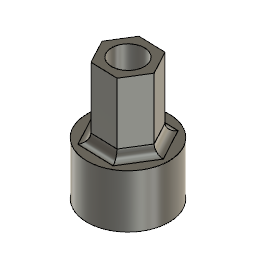
tt_motor_axle_adapter_6mm (Autodesk Fusion 360 design; units mm, degrees)
part number: 2026-02-17-20-52-45-499
Autodesk Fusion 360 part; units mm, degrees
sketch "Skizze1" plane through (0, 0, 0) normal (0, 0, 1) x (1, 0, 0)
  circle A0 centre (0, 0) radius 2.8
  circle A1 centre (0, 0) radius 5
  line L0 (1.95, -2.0094) -> (-1.95, -2.0094)
  line L1 (-1.95, -2.0094) -> (-1.95, 2.0094)
  line L2 (-1.95, 2.0094) -> (1.95, 2.0094)
  line L3 (1.95, 2.0094) -> (1.95, -2.0094)
  line L4 (1.95, -2.0094) -> (-1.95, 2.0094) construction
  line L5 (-1.95, -2.0094) -> (1.95, 2.0094) construction
  dimension "d1" = 5.6
  dimension "d2" = 10
  dimension "d3" = 3.9
  constraint coincident A0.centre A1.centre
  constraint horizontal L0
  constraint perpendicular L0 L1
  constraint parallel L0 L2
  constraint parallel L1 L3
  constraint coincident L4 A0.centre
  constraint coincident L5 A0.centre
  constraint coincident A0 L1.end
  measures "d1" diameter of A0
  measures "d2" diameter of A1
  measures "d3" distance of L1.end L2.end
extrude "Extrusion1" add sketch "Skizze1" along normal blind 6.5 contours A0 L3 | A0 L1 | A1 makes body 1
ref_plane "Arbeitsebene1" through (0, 0, 6.5) normal (0, 0, 1) x (1, 0, 0)
sketch "Skizze2" plane through (0, 0, 6.5) normal (0, 0, 1) x (1, 0, 0)
  line L0 (-3.2893, 0.101) -> (-1.7322, -2.7981)
  line L1 (-1.7322, -2.7981) -> (1.5572, -2.8992)
  line L2 (1.5572, -2.8992) -> (3.2893, -0.101)
  line L3 (3.2893, -0.101) -> (1.7322, 2.7981)
  line L4 (1.7322, 2.7981) -> (-1.5572, 2.8992)
  line L5 (-1.5572, 2.8992) -> (-3.2893, 0.101)
  dimension "d7" = 2.85
  measures "d7" distance of origin L5
extrude "Extrusion2" add sketch "Skizze2" along normal blind 10.5 separate body makes body 2
sketch "Skizze3" plane through (0, 0, 17) normal (0, 0, 1) x (-1, 0, 0)
  line L0 (1.5572, -2.8992) -> (3.2893, -0.101)
  line L1 (3.2893, -0.101) -> (1.7322, 2.7981)
  line L2 (1.7322, 2.7981) -> (-1.5572, 2.8992)
  line L3 (-1.5572, 2.8992) -> (-3.2893, 0.101)
  line L4 (-3.2893, 0.101) -> (-1.7322, -2.7981)
  line L5 (-1.7322, -2.7981) -> (1.5572, -2.8992)
  circle A0 centre (0, 0) radius 2
  dimension "d10" = 4
  constraint coincident A0.centre origin
  measures "d10" diameter of A0
extrude "Extrusion3" cut sketch "Skizze3" against normal blind 10.5 contours A0 bodies 2
combine "Kombinieren1" operation add target body 1 tool bodies 2
fillet "Abrundung1" radius 1 6 edges at (2.4233, -1.5001, 6.5) (2.5108, 1.3485, 6.5) (0.0875, 2.8487, 6.5) (-0.0875, -2.8487, 6.5) (-2.5108, -1.3485, 6.5) (-2.4233, 1.5001, 6.5) on bodies 1
extrude "Extrusion4" cut 1 faces at (-0.1082, -2.5639, 17) along direction (0, 0, -1) blind 2 on bodies 1 bodies 1
equation "d7 = ( 5.7 / 2 ) * 1 mm"
